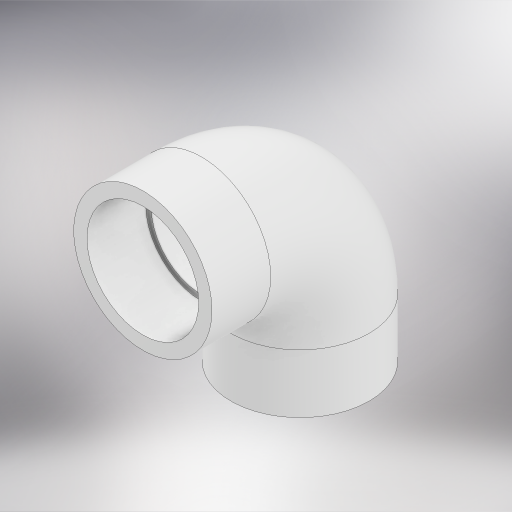
# Autodesk Inventor part: Codo
Saved by Autodesk Inventor 2023 (Build 270158000, 158)
## iProperties
Created: 2023-06-15
Part Number: Codo
Material: PVC, no plastificado
Document SubType Name: Modeling
Designer: Braya
Density: 1.29 g/cm^3
Appearance: Suave - Blanco
Author: Braya
Autodesk Inventor part; units mm, degrees
ref_plane "YZ Plane" through (0, 0, 0) normal (1, 0, 0) x (0, 1, 0)
ref_plane "XZ Plane" through (0, 0, 0) normal (0, 1, 0) x (-1, 0, 0)
ref_plane "XY Plane" through (0, 0, 0) normal (0, 0, 1) x (1, 0, 0)
sketch "Boceto6" plane through (0, 0, 0) normal (0, 1, 0) x (-1, 0, 0)
  line L0 (0, 0) -> (33, 0)
  line L1 (33, 0) -> (33, -40)
  line L2 (33, -40) -> (0, -40)
  line L3 (0, -40) -> (0, 0)
  line L4 (16.5, -40) -> (16.5, -23.5)
  circle A0 centre (16.5, -23.5) radius 16.5
  dimension "d12" = 33
  dimension "d13" = 40
  dimension "d14" = 16.5
  constraints: 10 end point, 2 parallel, 1 centre point, 1 coincident, 1 horizontal, 1 midpoint, 1 perpendicular, 1 tangent, 1 vertical
  measures "d12" distance of L1.end L2.end
  measures "d13" distance of L0.end L1.end
  measures "d14" distance of L4.start L4.end
sketch "Boceto7" plane through (0, 0, 0) normal (0, 0, 1) x (1, 0, 0)
  line L0 (0, 0) -> (-33, 0)
  line L1 (-33, 0) -> (-33, 40)
  line L2 (-33, 40) -> (0, 40)
  line L3 (0, 40) -> (0, 0)
  line L4 (-16.5, 40) -> (-16.5, 23.5)
  circle A0 centre (-16.5, 23.5) radius 16.5
  dimension "d15" = 33
  dimension "d16" = 40
  dimension "d17" = 16.5
  constraints: 10 end point, 2 parallel, 1 coincident, 1 horizontal, 1 midpoint, 1 perpendicular, 1 vertical, 1 vertical alignment, 2 other
  measures "d15" distance of L1.end L2.end
  measures "d16" distance of L0.end L1.end
  measures "d17" distance of L4.start L4.end
revolve "Revolución1" add sketch "Boceto7" angle 90 about axis through (0, 0, 0) along (-1, 0, 0) contours A0
sketch "Boceto8" plane through (-16.5, 23.5, 0) normal (0, 0, 1) x (1, 0, 0)
  circle A0 centre (0, 0) radius 16.5
  circle A1 centre (0, 0) radius 13.325
  point P0 (16.5, -23.5)
  dimension "d19" = 26.65
  constraints: 2 centre point, 1 coincident
  measures "d19" diameter of A1
extrude "Extrusión4" add sketch "Boceto8" along normal blind 14
sketch "Boceto9" plane through (-16.5, 0, -23.5) normal (0, -1, 0) x (1, 0, 0)
  circle A0 centre (0, 0) radius 16.5
  circle A1 centre (0, 0) radius 13.325
  point P0 (16.5, 23.5)
  dimension "d22" = 26.65
  constraints: 2 centre point, 1 coincident
  measures "d22" diameter of A1
extrude "Extrusión5" add sketch "Boceto9" along normal blind 14
sketch "Boceto10" plane through (-16.5, 23.5, 0) normal (0, 0, 1) x (1, 0, 0)
  circle A0 centre (0, 0) radius 12
  point P0 (16.5, -23.5)
  dimension "d25" = 24
  constraints: 1 centre point
  measures "d25" diameter of A0
revolve "Revolución2" cut sketch "Boceto10" angle 90 about axis through (0, 0, 0) along (-1, 0, 0)
